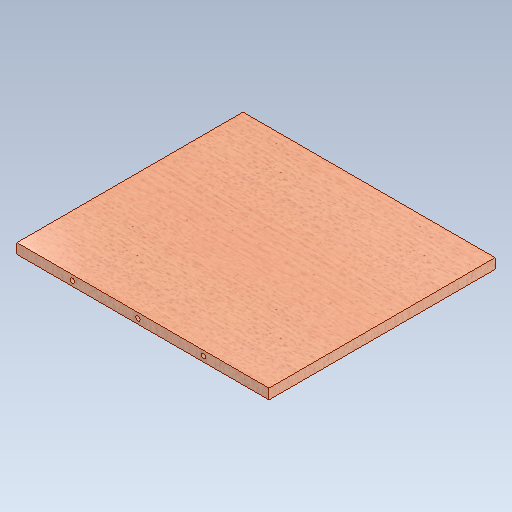
# Autodesk Inventor part: BaseCajoneras
Saved by Autodesk Inventor 2020.3 (Build 243373000, 373)
## iProperties
Created: 2020-10-30
Part Number: BaseCajoneras
Material: Madera (roble)
Document SubType Name: Modeling
Designer: codig
Density: 0.76 g/cm^3
Appearance: Roble blanco - Natural brillo medio
Author: codig
Autodesk Inventor part; units mm, degrees
ref_plane "YZ Plane" through (0, 0, 0) normal (1, 0, 0) x (0, 1, 0)
ref_plane "XZ Plane" through (0, 0, 0) normal (0, 1, 0) x (-1, 0, 0)
ref_plane "XY Plane" through (0, 0, 0) normal (0, 0, 1) x (1, 0, 0)
sketch "Boceto1" plane through (0, 0, 0) normal (0, 1, 0) x (-1, 0, 0)
  line L0 (100, -100) -> (546, -100)
  line L1 (546, -100) -> (546, -500)
  line L2 (546, -500) -> (100, -500)
  line L3 (100, -500) -> (100, -100)
  point P0 (0, 0)
  constraints: 8 end point, 2 parallel, 1 horizontal, 1 perpendicular
extrude "Extrusión1" add sketch "Boceto1" along normal blind 18
sketch "Boceto2" plane through (-546, 0, -100) normal (0, 0, 1) x (1, 0, 0)
  line L0 (446, 0) -> (446, 18) projected
  circle A0 centre (330, 9) radius 4
  circle A1 centre (214, 9) radius 4
  circle A2 centre (98, 9) radius 4
  point P0 (546, 0)
  constraints: 3 centre point
hole "Agujero1" at (-216, 9, -100) at (-332, 9, -100) at (-448, 9, -100) direction (0, 0, -1) diameter 8 depth 35
sketch "Boceto3" plane through (-100, 0, -500) normal (0, 0, -1) x (-1, 0, 0)
  line L0 (0, 0) -> (0, 18) projected
  circle A0 centre (116, 9) radius 4 projected
  circle A1 centre (116, 9) radius 4
  circle A2 centre (232, 9) radius 4 projected
  circle A3 centre (232, 9) radius 4
  circle A4 centre (348, 9) radius 4 projected
  circle A5 centre (348, 9) radius 4
  point P0 (-100, 0)
  constraints: 3 centre point, 2 coincident
hole "Agujero2" at (-216, 9, -500) at (-332, 9, -500) at (-448, 9, -500) direction (0, 0, 1) diameter 8 depth 35
